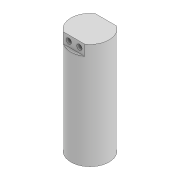
# Autodesk Inventor part: link1
Saved by Autodesk Inventor 2022 (Build 260153000, 153)
## iProperties
Created: 2022-03-09
Part Number: link1
Material: Generic
Document SubType Name: Modeling
Designer: piers
Density: 1 g/cm^3
Appearance: Default
Author: piers
Autodesk Inventor part; units mm, degrees
ref_plane "YZ Plane" through (0, 0, 0) normal (1, 0, 0) x (0, 1, 0)
ref_plane "XZ Plane" through (0, 0, 0) normal (0, 1, 0) x (-1, 0, 0)
ref_plane "XY Plane" through (0, 0, 0) normal (0, 0, 1) x (1, 0, 0)
sketch "Sketch1" plane through (0, 0, 0) normal (0, 1, 0) x (-1, 0, 0)
  circle A0 centre (0, 0) radius 18
  dimension "d0" = 36
  constraints: 1 centre point, 1 coincident
  measures "d0" diameter of A0
extrude "Extrusion1" add sketch "Sketch1" along normal blind 100
sketch "Sketch3" plane through (0, 100, 0) normal (0, 1, 0) x (1, 0, 0)
  circle A0 centre (0, 0) radius 18 projected
  line L0 (-10, 14.9666) -> (10, 14.9666)
  circle A1 centre (0, 0) radius 18 projected
  line L1 (0, 0) -> (10, 0)
  line L2 (-10, -14.9666) -> (10, -14.9666)
  point P0 (0, 14.9666)
  point P1 (10, 14.9666)
  point P2 (10, -14.9666)
  dimension "d6" = 20
  constraints: 6 end point, 2 symmetric about line, 1 horizontal, 1 horizontal alignment, 1 midpoint, 1 point on circle, 2 other
  measures "d6" distance of L0.start L0.end
extrude "Extrusion3" cut sketch "Sketch3" against normal blind 10 contours L0 A0 | A0 L2
sketch "Sketch4" plane through (10, 100, -14.9666) normal (0, 0, -1) x (-1, 0, 0)
  arc A0 (6.5, -7) -> (3.5, -7) centre (5, -5) ccw projected
  arc A1 (16.5, -7) -> (13.5, -7) centre (15, -5) ccw projected
  circle A2 centre (5, -5) radius 2.5
  circle A3 centre (15, -5) radius 2.5
  point P0 (10, -100)
  point P1 (3.5, -7)
  point P2 (6.5, -7)
  point P3 (13.5, -7)
  point P4 (16.5, -7)
  constraints: 2 centre point, 2 coincident, 2 concentric
extrude "Extrusion4" cut sketch "Sketch4" against normal through all
sketch "Sketch5" plane through (0, 0, 0) normal (0, -1, 0) x (1, 0, 0)
  circle A0 centre (13.5, 0) radius 1.5
  circle A1 centre (0, 13.5) radius 1.5
  circle A2 centre (-13.5, 0) radius 1.5
  circle A3 centre (0, -13.5) radius 1.5
  point P0 (0, 0)
  dimension "d11" = 3
  dimension "d12" = 13.5
  dimension "d15" = 360
  constraints: 4 centre point, 9 other
  measures "d11" diameter of A0
  measures "d12" distance of point (0, 0) A0.centre
extrude "Extrusion5" cut sketch "Sketch5" against normal blind 8
body "Solid1"
